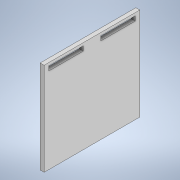
# Autodesk Inventor part: Long_Piece_Final
Saved by Autodesk Inventor 2022 (Build 260153000, 153)
## iProperties
Created: 2023-01-11
Part Number: Long_Piece_Final
Material: Generic
Document SubType Name: Modeling
Designer: s151859
Density: 1 g/cm^3
Appearance: Default
Author: s151859
Autodesk Inventor part; units mm, degrees
ref_plane "YZ Plane" through (0, 0, 0) normal (1, 0, 0) x (0, 1, 0)
ref_plane "XZ Plane" through (0, 0, 0) normal (0, 1, 0) x (-1, 0, 0)
ref_plane "XY Plane" through (0, 0, 0) normal (0, 0, 1) x (1, 0, 0)
sketch "Sketch1" plane through (0, 0, 0) normal (0, 1, 0) x (-1, 0, 0)
  line L0 (38.0427, 88.9138) -> (30.4227, 88.9138)
  line L1 (30.4227, 88.9138) -> (30.4227, -94.6012)
  line L2 (30.4227, -94.6012) -> (38.0427, -94.6012)
  line L3 (38.0427, -94.6012) -> (38.0427, 88.9138)
  point P0 (0, 0)
  dimension "d0" = 183.515
  dimension "d1" = 7.62
  constraints: 8 end point, 2 parallel, 1 horizontal, 1 perpendicular
  measures "d0" distance of L2.end L0.start
  measures "d1" distance of L0.start L0.end
extrude "Extrusion1" add sketch "Sketch1" along normal blind 177.8
sketch "Sketch2" plane through (-30.4227, 0, 88.9138) normal (1, 0, 0) x (0, 0, -1)
  line L0 (8.89, 172.72) -> (74.93, 172.72)
  line L1 (74.93, 172.72) -> (74.93, 163.83)
  line L2 (74.93, 163.83) -> (8.89, 163.83)
  line L3 (8.89, 163.83) -> (8.89, 172.72)
  line L4 (108.585, 172.72) -> (174.625, 172.72)
  line L5 (174.625, 172.72) -> (174.625, 163.83)
  line L6 (174.625, 163.83) -> (108.585, 163.83)
  line L7 (108.585, 163.83) -> (108.585, 172.72)
  line L8 (0, 0) -> (0, 177.8) projected
  line L9 (183.515, 0) -> (183.515, 177.8) projected
  line L10 (0, 177.8) -> (183.515, 177.8) projected
  point P0 (88.9138, 0)
  dimension "d4" = 66.04
  dimension "d5" = 66.04
  dimension "d6" = 8.89
  dimension "d7" = 8.89
  dimension "d8" = 8.89
  dimension "d9" = 5.08
  constraints: 16 end point, 4 parallel, 2 horizontal, 2 perpendicular, 2 point on line
  measures "d4" distance of L1.end L2.end
  measures "d5" distance of L5.end L6.end
  measures "d6" distance of L6.end L4.start
  measures "d7" distance between parallel lines of L8 L3
  measures "d8" distance between parallel lines of L5 L9
  measures "d9" distance between parallel lines of L10 L4
extrude "Extrusion2" cut sketch "Sketch2" against normal blind 25.4
body "Solid1"
